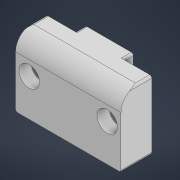
# Autodesk Inventor part: USB Clamp
Saved by Autodesk Inventor 2022 (Build 260153000, 153)
## iProperties
Created: 2021-07-20
Part Number: USB Clamp
Material: Generic
Document SubType Name: Modeling
Designer: trl121
Density: 1 g/cm^3
Appearance: Default
Author: trl121
Autodesk Inventor part; units mm, degrees
ref_plane "YZ Plane" through (0, 0, 0) normal (1, 0, 0) x (0, 1, 0)
ref_plane "XZ Plane" through (0, 0, 0) normal (0, 1, 0) x (-1, 0, 0)
ref_plane "Work Plane2" through (91.1943, 0, -5.3369) normal (0, 1, 0) x (0, 0, -1)
sketch "Sketch1" plane through (91.1943, 0, -5.3369) normal (0, 1, 0) x (0, 0, -1)
  arc A0 (2.2831, 81.0343) -> (1.0131, 82.3043) centre (1.0131, 81.0343) ccw construction
  line L0 (-5.3369, 82.3043) -> (1.0131, 82.3043) construction
  line L1 (2.2831, 81.0343) -> (2.2831, 68.3343) construction
  arc A1 (1.0131, 67.0643) -> (2.2831, 68.3343) centre (1.0131, 68.3343) ccw construction
  line L2 (1.0131, 67.0643) -> (-5.3369, 67.0643) construction
  line L3 (-5.3369, 67.0643) -> (-5.3369, 58.1743) construction
  line L4 (-5.3369, 91.1943) -> (-5.3369, 82.3043) construction
  line L5 (-5.3369, 58.1743) -> (-12.9569, 58.1743) construction
  line L6 (-12.9569, 91.1943) -> (-5.3369, 91.1943) construction
  line L7 (-18.0369, 58.1743) -> (-12.9569, 58.1743) construction
  line L8 (-12.9569, 91.1943) -> (-18.0369, 91.1943) construction
  line L9 (-18.0369, 58.3743) -> (-8.5119, 58.3743)
  line L10 (-8.5119, 58.3743) -> (-8.5119, 67.2643)
  line L11 (-8.5119, 67.2643) -> (-5.3369, 67.2643)
  line L12 (-18.0369, 58.3743) -> (-18.0369, 90.9943)
  line L13 (-18.0369, 90.9943) -> (-8.5119, 90.9943)
  line L14 (-8.5119, 90.9943) -> (-8.5119, 82.1043)
  line L15 (-8.5119, 82.1043) -> (-5.3369, 82.1043)
  line L16 (-18.0369, 74.6843) -> (-5.3369, 74.6843) construction
  arc A2 (-0.2019, 77.5293) -> (-2.8519, 77.5293) centre (-1.5269, 77.5293) ccw construction
  line L17 (-2.8519, 71.8393) -> (-2.8519, 77.5293) construction
  arc A3 (-2.8519, 71.8393) -> (-0.2019, 71.8393) centre (-1.5269, 71.8393) ccw construction
  line L18 (-0.2019, 77.5293) -> (-0.2019, 71.8393) construction
  line L19 (-1.5269, 71.8393) -> (-1.5269, 77.5293) construction
  line L20 (-5.3369, 67.2643) -> (-5.3369, 82.1043)
  line L21 (-18.0369, 58.1743) -> (-18.0369, 91.1943) construction
  dimension "d0" = 0.2
  dimension "d1" = 0.2
  dimension "d2" = 0.2
  dimension "d3" = 3.175
  constraints: 20 end point, 6 perpendicular, 2 collinear, 2 horizontal, 2 vertical, 2 vertical alignment, 1 midpoint, 2 other
  measures "d0" distance between parallel lines of L2 L11
  measures "d1" distance between parallel lines of L15 L0
  measures "d2" distance between parallel lines of L5 L9
  measures "d3" distance between parallel lines of L3 L10
extrude "Main Body" add sketch "Sketch1" against normal blind 21.082
sketch "Sketch2" plane through (0.2, 0, 12.7) normal (0, 0, 1) x (1, 0, 0)
  circle A0 centre (28.375, -9.525) radius 1.6 projected
  circle A1 centre (4.245, -9.525) radius 1.6 projected
  point P0 (-0.2, 0)
extrude "M3 Bolt" cut sketch "Sketch2" against normal up to next
sketch "Sketch3" plane through (0.2, 0, 12.7) normal (0, 0, 1) x (1, 0, 0)
  circle A0 centre (28.375, -9.525) radius 1.6 construction
  circle A1 centre (28.375, -9.525) radius 3.175
  circle A2 centre (4.245, -9.525) radius 1.6 construction
  circle A3 centre (4.245, -9.525) radius 3.175
  point P0 (-0.2, 0)
  dimension "d9" = 6.35
  constraints: 2 centre point, 2 coincident, 1 equal radius
  measures "d9" diameter of A1
extrude "M3 Bolt Head" cut sketch "Sketch3" against normal blind 3.81
sketch "Sketch4" plane through (23.93, 0, 0) normal (0, 0, -1) x (-1, 0, 0)
  line L0 (0.689, -2.032) -> (1.959, -2.032)
  line L1 (1.959, -2.032) -> (1.959, -0.762)
  line L2 (1.959, -0.762) -> (0.689, -0.762)
  line L3 (0.689, -0.762) -> (0.689, -2.032)
  line L4 (0, 0) -> (14.84, 0) construction
  line L5 (0, 0) -> (0, -21.082) construction
  line L6 (14.84, -21.082) -> (0, -21.082) construction
  line L7 (14.84, 0) -> (14.84, -21.082) construction
  line L8 (0, 0) -> (0, -21.082) construction
  line L9 (0, -21.082) -> (14.84, 0) construction
  line L10 (1.959, -3.556) -> (1.959, -2.286)
  line L11 (1.959, -2.286) -> (0.689, -2.286)
  line L12 (0.689, -2.286) -> (0.689, -3.556)
  line L13 (0.689, -3.556) -> (1.959, -3.556)
  line L14 (1.959, -5.08) -> (1.959, -3.81)
  line L15 (1.959, -3.81) -> (0.689, -3.81)
  line L16 (0.689, -3.81) -> (0.689, -5.08)
  line L17 (0.689, -5.08) -> (1.959, -5.08)
  line L18 (1.959, -6.604) -> (1.959, -5.334)
  line L19 (1.959, -5.334) -> (0.689, -5.334)
  line L20 (0.689, -5.334) -> (0.689, -6.604)
  line L21 (0.689, -6.604) -> (1.959, -6.604)
  line L22 (1.959, -8.128) -> (1.959, -6.858)
  line L23 (1.959, -6.858) -> (0.689, -6.858)
  line L24 (0.689, -6.858) -> (0.689, -8.128)
  line L25 (0.689, -8.128) -> (1.959, -8.128)
  line L26 (1.959, -9.652) -> (1.959, -8.382)
  line L27 (1.959, -8.382) -> (0.689, -8.382)
  line L28 (0.689, -8.382) -> (0.689, -9.652)
  line L29 (0.689, -9.652) -> (1.959, -9.652)
  line L30 (1.959, -11.176) -> (1.959, -9.906)
  line L31 (1.959, -9.906) -> (0.689, -9.906)
  line L32 (0.689, -9.906) -> (0.689, -11.176)
  line L33 (0.689, -11.176) -> (1.959, -11.176)
  line L34 (1.959, -12.7) -> (1.959, -11.43)
  line L35 (1.959, -11.43) -> (0.689, -11.43)
  line L36 (0.689, -11.43) -> (0.689, -12.7)
  line L37 (0.689, -12.7) -> (1.959, -12.7)
  line L38 (1.959, -14.224) -> (1.959, -12.954)
  line L39 (1.959, -12.954) -> (0.689, -12.954)
  line L40 (0.689, -12.954) -> (0.689, -14.224)
  line L41 (0.689, -14.224) -> (1.959, -14.224)
  line L42 (1.959, -15.748) -> (1.959, -14.478)
  line L43 (1.959, -14.478) -> (0.689, -14.478)
  line L44 (0.689, -14.478) -> (0.689, -15.748)
  line L45 (0.689, -15.748) -> (1.959, -15.748)
  line L46 (1.959, -17.272) -> (1.959, -16.002)
  line L47 (1.959, -16.002) -> (0.689, -16.002)
  line L48 (0.689, -16.002) -> (0.689, -17.272)
  line L49 (0.689, -17.272) -> (1.959, -17.272)
  line L50 (1.959, -18.796) -> (1.959, -17.526)
  line L51 (1.959, -17.526) -> (0.689, -17.526)
  line L52 (0.689, -17.526) -> (0.689, -18.796)
  line L53 (0.689, -18.796) -> (1.959, -18.796)
  line L54 (3.483, -2.032) -> (3.483, -0.762)
  line L55 (3.483, -0.762) -> (2.213, -0.762)
  line L56 (2.213, -0.762) -> (2.213, -2.032)
  line L57 (2.213, -2.032) -> (3.483, -2.032)
  line L58 (3.483, -3.556) -> (3.483, -2.286)
  line L59 (3.483, -2.286) -> (2.213, -2.286)
  line L60 (2.213, -2.286) -> (2.213, -3.556)
  line L61 (2.213, -3.556) -> (3.483, -3.556)
  line L62 (3.483, -5.08) -> (3.483, -3.81)
  line L63 (3.483, -3.81) -> (2.213, -3.81)
  line L64 (2.213, -3.81) -> (2.213, -5.08)
  line L65 (2.213, -5.08) -> (3.483, -5.08)
  line L66 (3.483, -6.604) -> (3.483, -5.334)
  line L67 (3.483, -5.334) -> (2.213, -5.334)
  line L68 (2.213, -5.334) -> (2.213, -6.604)
  line L69 (2.213, -6.604) -> (3.483, -6.604)
  line L70 (3.483, -8.128) -> (3.483, -6.858)
  line L71 (3.483, -6.858) -> (2.213, -6.858)
  line L72 (2.213, -6.858) -> (2.213, -8.128)
  line L73 (2.213, -8.128) -> (3.483, -8.128)
  line L74 (3.483, -9.652) -> (3.483, -8.382)
  line L75 (3.483, -8.382) -> (2.213, -8.382)
  line L76 (2.213, -8.382) -> (2.213, -9.652)
  line L77 (2.213, -9.652) -> (3.483, -9.652)
  line L78 (3.483, -11.176) -> (3.483, -9.906)
  line L79 (3.483, -9.906) -> (2.213, -9.906)
  line L80 (2.213, -9.906) -> (2.213, -11.176)
  line L81 (2.213, -11.176) -> (3.483, -11.176)
  line L82 (3.483, -12.7) -> (3.483, -11.43)
  line L83 (3.483, -11.43) -> (2.213, -11.43)
  line L84 (2.213, -11.43) -> (2.213, -12.7)
  line L85 (2.213, -12.7) -> (3.483, -12.7)
  line L86 (3.483, -14.224) -> (3.483, -12.954)
  line L87 (3.483, -12.954) -> (2.213, -12.954)
  line L88 (2.213, -12.954) -> (2.213, -14.224)
  line L89 (2.213, -14.224) -> (3.483, -14.224)
  line L90 (3.483, -15.748) -> (3.483, -14.478)
  line L91 (3.483, -14.478) -> (2.213, -14.478)
  line L92 (2.213, -14.478) -> (2.213, -15.748)
  line L93 (2.213, -15.748) -> (3.483, -15.748)
  line L94 (3.483, -17.272) -> (3.483, -16.002)
  line L95 (3.483, -16.002) -> (2.213, -16.002)
  line L96 (2.213, -16.002) -> (2.213, -17.272)
  line L97 (2.213, -17.272) -> (3.483, -17.272)
  line L98 (3.483, -18.796) -> (3.483, -17.526)
  line L99 (3.483, -17.526) -> (2.213, -17.526)
  line L100 (2.213, -17.526) -> (2.213, -18.796)
  line L101 (2.213, -18.796) -> (3.483, -18.796)
  line L102 (5.007, -2.032) -> (5.007, -0.762)
  line L103 (5.007, -0.762) -> (3.737, -0.762)
  line L104 (3.737, -0.762) -> (3.737, -2.032)
  line L105 (3.737, -2.032) -> (5.007, -2.032)
  line L106 (5.007, -3.556) -> (5.007, -2.286)
  line L107 (5.007, -2.286) -> (3.737, -2.286)
  line L108 (3.737, -2.286) -> (3.737, -3.556)
  line L109 (3.737, -3.556) -> (5.007, -3.556)
  line L110 (5.007, -5.08) -> (5.007, -3.81)
  line L111 (5.007, -3.81) -> (3.737, -3.81)
  line L112 (3.737, -3.81) -> (3.737, -5.08)
  line L113 (3.737, -5.08) -> (5.007, -5.08)
  line L114 (5.007, -6.604) -> (5.007, -5.334)
  line L115 (5.007, -5.334) -> (3.737, -5.334)
  line L116 (3.737, -5.334) -> (3.737, -6.604)
  line L117 (3.737, -6.604) -> (5.007, -6.604)
  line L118 (5.007, -8.128) -> (5.007, -6.858)
  line L119 (5.007, -6.858) -> (3.737, -6.858)
  line L120 (3.737, -6.858) -> (3.737, -8.128)
  line L121 (3.737, -8.128) -> (5.007, -8.128)
  line L122 (5.007, -9.652) -> (5.007, -8.382)
  line L123 (5.007, -8.382) -> (3.737, -8.382)
  line L124 (3.737, -8.382) -> (3.737, -9.652)
  line L125 (3.737, -9.652) -> (5.007, -9.652)
  line L126 (5.007, -11.176) -> (5.007, -9.906)
  line L127 (5.007, -9.906) -> (3.737, -9.906)
  line L128 (3.737, -9.906) -> (3.737, -11.176)
  line L129 (3.737, -11.176) -> (5.007, -11.176)
  line L130 (5.007, -12.7) -> (5.007, -11.43)
  line L131 (5.007, -11.43) -> (3.737, -11.43)
  line L132 (3.737, -11.43) -> (3.737, -12.7)
  line L133 (3.737, -12.7) -> (5.007, -12.7)
  line L134 (5.007, -14.224) -> (5.007, -12.954)
  line L135 (5.007, -12.954) -> (3.737, -12.954)
  line L136 (3.737, -12.954) -> (3.737, -14.224)
  line L137 (3.737, -14.224) -> (5.007, -14.224)
  line L138 (5.007, -15.748) -> (5.007, -14.478)
  line L139 (5.007, -14.478) -> (3.737, -14.478)
  line L140 (3.737, -14.478) -> (3.737, -15.748)
  line L141 (3.737, -15.748) -> (5.007, -15.748)
  line L142 (5.007, -17.272) -> (5.007, -16.002)
  line L143 (5.007, -16.002) -> (3.737, -16.002)
  line L144 (3.737, -16.002) -> (3.737, -17.272)
  line L145 (3.737, -17.272) -> (5.007, -17.272)
  line L146 (5.007, -18.796) -> (5.007, -17.526)
  line L147 (5.007, -17.526) -> (3.737, -17.526)
  line L148 (3.737, -17.526) -> (3.737, -18.796)
  line L149 (3.737, -18.796) -> (5.007, -18.796)
  line L150 (6.531, -2.032) -> (6.531, -0.762)
  line L151 (6.531, -0.762) -> (5.261, -0.762)
  line L152 (5.261, -0.762) -> (5.261, -2.032)
  line L153 (5.261, -2.032) -> (6.531, -2.032)
  line L154 (6.531, -3.556) -> (6.531, -2.286)
  line L155 (6.531, -2.286) -> (5.261, -2.286)
  line L156 (5.261, -2.286) -> (5.261, -3.556)
  line L157 (5.261, -3.556) -> (6.531, -3.556)
  line L158 (6.531, -5.08) -> (6.531, -3.81)
  line L159 (6.531, -3.81) -> (5.261, -3.81)
  line L160 (5.261, -3.81) -> (5.261, -5.08)
  line L161 (5.261, -5.08) -> (6.531, -5.08)
  line L162 (6.531, -6.604) -> (6.531, -5.334)
  line L163 (6.531, -5.334) -> (5.261, -5.334)
  line L164 (5.261, -5.334) -> (5.261, -6.604)
  line L165 (5.261, -6.604) -> (6.531, -6.604)
  line L166 (6.531, -8.128) -> (6.531, -6.858)
  line L167 (6.531, -6.858) -> (5.261, -6.858)
  line L168 (5.261, -6.858) -> (5.261, -8.128)
  line L169 (5.261, -8.128) -> (6.531, -8.128)
  line L170 (6.531, -9.652) -> (6.531, -8.382)
  line L171 (6.531, -8.382) -> (5.261, -8.382)
  line L172 (5.261, -8.382) -> (5.261, -9.652)
  line L173 (5.261, -9.652) -> (6.531, -9.652)
  line L174 (6.531, -11.176) -> (6.531, -9.906)
  line L175 (6.531, -9.906) -> (5.261, -9.906)
  line L176 (5.261, -9.906) -> (5.261, -11.176)
  line L177 (5.261, -11.176) -> (6.531, -11.176)
  line L178 (6.531, -12.7) -> (6.531, -11.43)
  line L179 (6.531, -11.43) -> (5.261, -11.43)
  line L180 (5.261, -11.43) -> (5.261, -12.7)
  line L181 (5.261, -12.7) -> (6.531, -12.7)
  line L182 (6.531, -14.224) -> (6.531, -12.954)
  line L183 (6.531, -12.954) -> (5.261, -12.954)
  line L184 (5.261, -12.954) -> (5.261, -14.224)
  line L185 (5.261, -14.224) -> (6.531, -14.224)
  line L186 (6.531, -15.748) -> (6.531, -14.478)
  line L187 (6.531, -14.478) -> (5.261, -14.478)
  line L188 (5.261, -14.478) -> (5.261, -15.748)
  line L189 (5.261, -15.748) -> (6.531, -15.748)
  line L190 (6.531, -17.272) -> (6.531, -16.002)
  line L191 (6.531, -16.002) -> (5.261, -16.002)
  line L192 (5.261, -16.002) -> (5.261, -17.272)
  line L193 (5.261, -17.272) -> (6.531, -17.272)
  line L194 (6.531, -18.796) -> (6.531, -17.526)
  line L195 (6.531, -17.526) -> (5.261, -17.526)
  line L196 (5.261, -17.526) -> (5.261, -18.796)
  line L197 (5.261, -18.796) -> (6.531, -18.796)
  line L198 (8.055, -2.032) -> (8.055, -0.762)
  line L199 (8.055, -0.762) -> (6.785, -0.762)
  line L200 (6.785, -0.762) -> (6.785, -2.032)
  line L201 (6.785, -2.032) -> (8.055, -2.032)
  line L202 (8.055, -3.556) -> (8.055, -2.286)
  line L203 (8.055, -2.286) -> (6.785, -2.286)
  line L204 (6.785, -2.286) -> (6.785, -3.556)
  line L205 (6.785, -3.556) -> (8.055, -3.556)
  line L206 (8.055, -5.08) -> (8.055, -3.81)
  line L207 (8.055, -3.81) -> (6.785, -3.81)
  line L208 (6.785, -3.81) -> (6.785, -5.08)
  line L209 (6.785, -5.08) -> (8.055, -5.08)
  line L210 (8.055, -6.604) -> (8.055, -5.334)
  line L211 (8.055, -5.334) -> (6.785, -5.334)
  line L212 (6.785, -5.334) -> (6.785, -6.604)
  line L213 (6.785, -6.604) -> (8.055, -6.604)
  line L214 (8.055, -8.128) -> (8.055, -6.858)
  line L215 (8.055, -6.858) -> (6.785, -6.858)
  line L216 (6.785, -6.858) -> (6.785, -8.128)
  line L217 (6.785, -8.128) -> (8.055, -8.128)
  line L218 (8.055, -9.652) -> (8.055, -8.382)
  line L219 (8.055, -8.382) -> (6.785, -8.382)
  line L220 (6.785, -8.382) -> (6.785, -9.652)
  line L221 (6.785, -9.652) -> (8.055, -9.652)
  line L222 (8.055, -11.176) -> (8.055, -9.906)
  line L223 (8.055, -9.906) -> (6.785, -9.906)
  line L224 (6.785, -9.906) -> (6.785, -11.176)
  line L225 (6.785, -11.176) -> (8.055, -11.176)
  line L226 (8.055, -12.7) -> (8.055, -11.43)
  line L227 (8.055, -11.43) -> (6.785, -11.43)
  line L228 (6.785, -11.43) -> (6.785, -12.7)
  line L229 (6.785, -12.7) -> (8.055, -12.7)
  line L230 (8.055, -14.224) -> (8.055, -12.954)
  line L231 (8.055, -12.954) -> (6.785, -12.954)
  line L232 (6.785, -12.954) -> (6.785, -14.224)
  line L233 (6.785, -14.224) -> (8.055, -14.224)
  line L234 (8.055, -15.748) -> (8.055, -14.478)
  line L235 (8.055, -14.478) -> (6.785, -14.478)
  line L236 (6.785, -14.478) -> (6.785, -15.748)
  line L237 (6.785, -15.748) -> (8.055, -15.748)
  line L238 (8.055, -17.272) -> (8.055, -16.002)
  line L239 (8.055, -16.002) -> (6.785, -16.002)
  line L240 (6.785, -16.002) -> (6.785, -17.272)
  line L241 (6.785, -17.272) -> (8.055, -17.272)
  line L242 (8.055, -18.796) -> (8.055, -17.526)
  line L243 (8.055, -17.526) -> (6.785, -17.526)
  line L244 (6.785, -17.526) -> (6.785, -18.796)
  line L245 (6.785, -18.796) -> (8.055, -18.796)
  line L246 (9.579, -2.032) -> (9.579, -0.762)
  line L247 (9.579, -0.762) -> (8.309, -0.762)
  line L248 (8.309, -0.762) -> (8.309, -2.032)
  line L249 (8.309, -2.032) -> (9.579, -2.032)
  line L250 (9.579, -3.556) -> (9.579, -2.286)
  line L251 (9.579, -2.286) -> (8.309, -2.286)
  line L252 (8.309, -2.286) -> (8.309, -3.556)
  line L253 (8.309, -3.556) -> (9.579, -3.556)
  line L254 (9.579, -5.08) -> (9.579, -3.81)
  line L255 (9.579, -3.81) -> (8.309, -3.81)
  line L256 (8.309, -3.81) -> (8.309, -5.08)
  line L257 (8.309, -5.08) -> (9.579, -5.08)
  line L258 (9.579, -6.604) -> (9.579, -5.334)
  line L259 (9.579, -5.334) -> (8.309, -5.334)
  line L260 (8.309, -5.334) -> (8.309, -6.604)
  line L261 (8.309, -6.604) -> (9.579, -6.604)
  line L262 (9.579, -8.128) -> (9.579, -6.858)
  line L263 (9.579, -6.858) -> (8.309, -6.858)
  line L264 (8.309, -6.858) -> (8.309, -8.128)
  line L265 (8.309, -8.128) -> (9.579, -8.128)
  line L266 (9.579, -9.652) -> (9.579, -8.382)
  line L267 (9.579, -8.382) -> (8.309, -8.382)
  line L268 (8.309, -8.382) -> (8.309, -9.652)
  line L269 (8.309, -9.652) -> (9.579, -9.652)
  line L270 (9.579, -11.176) -> (9.579, -9.906)
  line L271 (9.579, -9.906) -> (8.309, -9.906)
  line L272 (8.309, -9.906) -> (8.309, -11.176)
  line L273 (8.309, -11.176) -> (9.579, -11.176)
  line L274 (9.579, -12.7) -> (9.579, -11.43)
  line L275 (9.579, -11.43) -> (8.309, -11.43)
  line L276 (8.309, -11.43) -> (8.309, -12.7)
  line L277 (8.309, -12.7) -> (9.579, -12.7)
  line L278 (9.579, -14.224) -> (9.579, -12.954)
  line L279 (9.579, -12.954) -> (8.309, -12.954)
  line L280 (8.309, -12.954) -> (8.309, -14.224)
  line L281 (8.309, -14.224) -> (9.579, -14.224)
  line L282 (9.579, -15.748) -> (9.579, -14.478)
  line L283 (9.579, -14.478) -> (8.309, -14.478)
  line L284 (8.309, -14.478) -> (8.309, -15.748)
  line L285 (8.309, -15.748) -> (9.579, -15.748)
  line L286 (9.579, -17.272) -> (9.579, -16.002)
  line L287 (9.579, -16.002) -> (8.309, -16.002)
  line L288 (8.309, -16.002) -> (8.309, -17.272)
  line L289 (8.309, -17.272) -> (9.579, -17.272)
  line L290 (9.579, -18.796) -> (9.579, -17.526)
  line L291 (9.579, -17.526) -> (8.309, -17.526)
  line L292 (8.309, -17.526) -> (8.309, -18.796)
  line L293 (8.309, -18.796) -> (9.579, -18.796)
  line L294 (11.103, -2.032) -> (11.103, -0.762)
  line L295 (11.103, -0.762) -> (9.833, -0.762)
  line L296 (9.833, -0.762) -> (9.833, -2.032)
  line L297 (9.833, -2.032) -> (11.103, -2.032)
  line L298 (11.103, -3.556) -> (11.103, -2.286)
  line L299 (11.103, -2.286) -> (9.833, -2.286)
  line L300 (9.833, -2.286) -> (9.833, -3.556)
  line L301 (9.833, -3.556) -> (11.103, -3.556)
  line L302 (11.103, -5.08) -> (11.103, -3.81)
  line L303 (11.103, -3.81) -> (9.833, -3.81)
  line L304 (9.833, -3.81) -> (9.833, -5.08)
  line L305 (9.833, -5.08) -> (11.103, -5.08)
  line L306 (11.103, -6.604) -> (11.103, -5.334)
  line L307 (11.103, -5.334) -> (9.833, -5.334)
  line L308 (9.833, -5.334) -> (9.833, -6.604)
  line L309 (9.833, -6.604) -> (11.103, -6.604)
  line L310 (11.103, -8.128) -> (11.103, -6.858)
  line L311 (11.103, -6.858) -> (9.833, -6.858)
  line L312 (9.833, -6.858) -> (9.833, -8.128)
  line L313 (9.833, -8.128) -> (11.103, -8.128)
  line L314 (11.103, -9.652) -> (11.103, -8.382)
  line L315 (11.103, -8.382) -> (9.833, -8.382)
  line L316 (9.833, -8.382) -> (9.833, -9.652)
  line L317 (9.833, -9.652) -> (11.103, -9.652)
  line L318 (11.103, -11.176) -> (11.103, -9.906)
  line L319 (11.103, -9.906) -> (9.833, -9.906)
  line L320 (9.833, -9.906) -> (9.833, -11.176)
  line L321 (9.833, -11.176) -> (11.103, -11.176)
  line L322 (11.103, -12.7) -> (11.103, -11.43)
  line L323 (11.103, -11.43) -> (9.833, -11.43)
  line L324 (9.833, -11.43) -> (9.833, -12.7)
  line L325 (9.833, -12.7) -> (11.103, -12.7)
  line L326 (11.103, -14.224) -> (11.103, -12.954)
  line L327 (11.103, -12.954) -> (9.833, -12.954)
  line L328 (9.833, -12.954) -> (9.833, -14.224)
  line L329 (9.833, -14.224) -> (11.103, -14.224)
  line L330 (11.103, -15.748) -> (11.103, -14.478)
  line L331 (11.103, -14.478) -> (9.833, -14.478)
  line L332 (9.833, -14.478) -> (9.833, -15.748)
  line L333 (9.833, -15.748) -> (11.103, -15.748)
  line L334 (11.103, -17.272) -> (11.103, -16.002)
  line L335 (11.103, -16.002) -> (9.833, -16.002)
  line L336 (9.833, -16.002) -> (9.833, -17.272)
  line L337 (9.833, -17.272) -> (11.103, -17.272)
  line L338 (11.103, -18.796) -> (11.103, -17.526)
  line L339 (11.103, -17.526) -> (9.833, -17.526)
  line L340 (9.833, -17.526) -> (9.833, -18.796)
  line L341 (9.833, -18.796) -> (11.103, -18.796)
  line L342 (12.627, -2.032) -> (12.627, -0.762)
  line L343 (12.627, -0.762) -> (11.357, -0.762)
  line L344 (11.357, -0.762) -> (11.357, -2.032)
  line L345 (11.357, -2.032) -> (12.627, -2.032)
  line L346 (12.627, -3.556) -> (12.627, -2.286)
  line L347 (12.627, -2.286) -> (11.357, -2.286)
  line L348 (11.357, -2.286) -> (11.357, -3.556)
  line L349 (11.357, -3.556) -> (12.627, -3.556)
  line L350 (12.627, -5.08) -> (12.627, -3.81)
  line L351 (12.627, -3.81) -> (11.357, -3.81)
  line L352 (11.357, -3.81) -> (11.357, -5.08)
  line L353 (11.357, -5.08) -> (12.627, -5.08)
  line L354 (12.627, -6.604) -> (12.627, -5.334)
  line L355 (12.627, -5.334) -> (11.357, -5.334)
  line L356 (11.357, -5.334) -> (11.357, -6.604)
  line L357 (11.357, -6.604) -> (12.627, -6.604)
  line L358 (12.627, -8.128) -> (12.627, -6.858)
  line L359 (12.627, -6.858) -> (11.357, -6.858)
  line L360 (11.357, -6.858) -> (11.357, -8.128)
  line L361 (11.357, -8.128) -> (12.627, -8.128)
  line L362 (12.627, -9.652) -> (12.627, -8.382)
  line L363 (12.627, -8.382) -> (11.357, -8.382)
  line L364 (11.357, -8.382) -> (11.357, -9.652)
  line L365 (11.357, -9.652) -> (12.627, -9.652)
  line L366 (12.627, -11.176) -> (12.627, -9.906)
  line L367 (12.627, -9.906) -> (11.357, -9.906)
  line L368 (11.357, -9.906) -> (11.357, -11.176)
  line L369 (11.357, -11.176) -> (12.627, -11.176)
  line L370 (12.627, -12.7) -> (12.627, -11.43)
  line L371 (12.627, -11.43) -> (11.357, -11.43)
  line L372 (11.357, -11.43) -> (11.357, -12.7)
  line L373 (11.357, -12.7) -> (12.627, -12.7)
  line L374 (12.627, -14.224) -> (12.627, -12.954)
  line L375 (12.627, -12.954) -> (11.357, -12.954)
  line L376 (11.357, -12.954) -> (11.357, -14.224)
  line L377 (11.357, -14.224) -> (12.627, -14.224)
  line L378 (12.627, -15.748) -> (12.627, -14.478)
  line L379 (12.627, -14.478) -> (11.357, -14.478)
  line L380 (11.357, -14.478) -> (11.357, -15.748)
  line L381 (11.357, -15.748) -> (12.627, -15.748)
  line L382 (12.627, -17.272) -> (12.627, -16.002)
  line L383 (12.627, -16.002) -> (11.357, -16.002)
  line L384 (11.357, -16.002) -> (11.357, -17.272)
  line L385 (11.357, -17.272) -> (12.627, -17.272)
  line L386 (12.627, -18.796) -> (12.627, -17.526)
  line L387 (12.627, -17.526) -> (11.357, -17.526)
  line L388 (11.357, -17.526) -> (11.357, -18.796)
  line L389 (11.357, -18.796) -> (12.627, -18.796)
  line L390 (14.151, -2.032) -> (14.151, -0.762)
  line L391 (14.151, -0.762) -> (12.881, -0.762)
  line L392 (12.881, -0.762) -> (12.881, -2.032)
  line L393 (12.881, -2.032) -> (14.151, -2.032)
  line L394 (14.151, -3.556) -> (14.151, -2.286)
  line L395 (14.151, -2.286) -> (12.881, -2.286)
  line L396 (12.881, -2.286) -> (12.881, -3.556)
  line L397 (12.881, -3.556) -> (14.151, -3.556)
  line L398 (14.151, -5.08) -> (14.151, -3.81)
  line L399 (14.151, -3.81) -> (12.881, -3.81)
  line L400 (12.881, -3.81) -> (12.881, -5.08)
  line L401 (12.881, -5.08) -> (14.151, -5.08)
  line L402 (14.151, -6.604) -> (14.151, -5.334)
  line L403 (14.151, -5.334) -> (12.881, -5.334)
  line L404 (12.881, -5.334) -> (12.881, -6.604)
  line L405 (12.881, -6.604) -> (14.151, -6.604)
  line L406 (14.151, -8.128) -> (14.151, -6.858)
  line L407 (14.151, -6.858) -> (12.881, -6.858)
  line L408 (12.881, -6.858) -> (12.881, -8.128)
  line L409 (12.881, -8.128) -> (14.151, -8.128)
  line L410 (14.151, -9.652) -> (14.151, -8.382)
  line L411 (14.151, -8.382) -> (12.881, -8.382)
  line L412 (12.881, -8.382) -> (12.881, -9.652)
  line L413 (12.881, -9.652) -> (14.151, -9.652)
  line L414 (14.151, -11.176) -> (14.151, -9.906)
  line L415 (14.151, -9.906) -> (12.881, -9.906)
  line L416 (12.881, -9.906) -> (12.881, -11.176)
  line L417 (12.881, -11.176) -> (14.151, -11.176)
  line L418 (14.151, -12.7) -> (14.151, -11.43)
  line L419 (14.151, -11.43) -> (12.881, -11.43)
  line L420 (12.881, -11.43) -> (12.881, -12.7)
  line L421 (12.881, -12.7) -> (14.151, -12.7)
  line L422 (14.151, -14.224) -> (14.151, -12.954)
  line L423 (14.151, -12.954) -> (12.881, -12.954)
  line L424 (12.881, -12.954) -> (12.881, -14.224)
  line L425 (12.881, -14.224) -> (14.151, -14.224)
  line L426 (14.151, -15.748) -> (14.151, -14.478)
  line L427 (14.151, -14.478) -> (12.881, -14.478)
  line L428 (12.881, -14.478) -> (12.881, -15.748)
  line L429 (12.881, -15.748) -> (14.151, -15.748)
  line L430 (14.151, -17.272) -> (14.151, -16.002)
  line L431 (14.151, -16.002) -> (12.881, -16.002)
  line L432 (12.881, -16.002) -> (12.881, -17.272)
  line L433 (12.881, -17.272) -> (14.151, -17.272)
  line L434 (14.151, -18.796) -> (14.151, -17.526)
  line L435 (14.151, -17.526) -> (12.881, -17.526)
  line L436 (12.881, -17.526) -> (12.881, -18.796)
  line L437 (12.881, -18.796) -> (14.151, -18.796)
  line L438 (1.959, -20.32) -> (1.959, -19.05)
  line L439 (1.959, -19.05) -> (0.689, -19.05)
  line L440 (0.689, -19.05) -> (0.689, -20.32)
  line L441 (0.689, -20.32) -> (1.959, -20.32)
  line L442 (3.483, -20.32) -> (3.483, -19.05)
  line L443 (3.483, -19.05) -> (2.213, -19.05)
  line L444 (2.213, -19.05) -> (2.213, -20.32)
  line L445 (2.213, -20.32) -> (3.483, -20.32)
  line L446 (5.007, -20.32) -> (5.007, -19.05)
  line L447 (5.007, -19.05) -> (3.737, -19.05)
  line L448 (3.737, -19.05) -> (3.737, -20.32)
  line L449 (3.737, -20.32) -> (5.007, -20.32)
  line L450 (6.531, -20.32) -> (6.531, -19.05)
  line L451 (6.531, -19.05) -> (5.261, -19.05)
  line L452 (5.261, -19.05) -> (5.261, -20.32)
  line L453 (5.261, -20.32) -> (6.531, -20.32)
  line L454 (8.055, -20.32) -> (8.055, -19.05)
  line L455 (8.055, -19.05) -> (6.785, -19.05)
  line L456 (6.785, -19.05) -> (6.785, -20.32)
  line L457 (6.785, -20.32) -> (8.055, -20.32)
  line L458 (9.579, -20.32) -> (9.579, -19.05)
  line L459 (9.579, -19.05) -> (8.309, -19.05)
  line L460 (8.309, -19.05) -> (8.309, -20.32)
  line L461 (8.309, -20.32) -> (9.579, -20.32)
  line L462 (11.103, -20.32) -> (11.103, -19.05)
  line L463 (11.103, -19.05) -> (9.833, -19.05)
  line L464 (9.833, -19.05) -> (9.833, -20.32)
  line L465 (9.833, -20.32) -> (11.103, -20.32)
  line L466 (12.627, -20.32) -> (12.627, -19.05)
  line L467 (12.627, -19.05) -> (11.357, -19.05)
  line L468 (11.357, -19.05) -> (11.357, -20.32)
  line L469 (11.357, -20.32) -> (12.627, -20.32)
  line L470 (14.151, -20.32) -> (14.151, -19.05)
  line L471 (14.151, -19.05) -> (12.881, -19.05)
  line L472 (12.881, -19.05) -> (12.881, -20.32)
  line L473 (12.881, -20.32) -> (14.151, -20.32)
  line L474 (0.689, -20.32) -> (14.151, -0.762) construction
  point P0 (23.93, 0)
  point P1 (7.42, -10.541)
  dimension "d13" = 1.27
  dimension "d16" = 1.524
  dimension "d19" = 1.524
  constraints: 940 end point, 2 collinear, 2 horizontal, 2 midpoint, 2 parallel, 2 perpendicular, 1 vertical, 926 other
  measures "d13" distance of L2.end L0.start
  measures "d16" distance of L0.end L10.start
  measures "d19" distance of L0.end L54.start
extrude "Bottom Grips" add sketch "Sketch4" along normal blind 25.4 draft -40
fillet "Fillets" radius 0.635 8 edges at (32.82, -21.082, 7.9375) (0.2, -21.082, 7.9375) (32.82, 0, 7.9375) (0.2, 0, 7.9375) (23.93, 0, 1.5875) (9.09, 0, 1.5875) (23.93, -21.082, 1.5875) (9.09, -21.082, 1.5875)
fillet "Fillets" radius 5.08 1 edges at (16.51, 0, 12.7)
equation "\"d1\" = d0"
body "Solid1"
